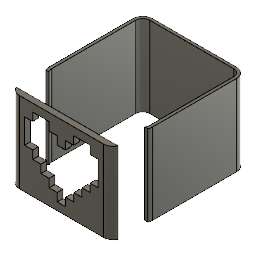
sides (Autodesk Fusion 360 design; units mm, degrees)
Autodesk Fusion 360 part; units mm, degrees
note: some values were not read from the file. Chosen so that the rebuilt part matches the saved one: which bodies a step acts on.
sketch "Sketch1" plane through (0, 0, 0) normal (0, 1, 0) x (1, 0, 0)
  line L0 (35.25, -35.25) -> (-35.25, -35.25)
  line L1 (-35.25, -35.25) -> (-35.25, 35.25)
  line L2 (-35.25, 35.25) -> (35.25, 35.25)
  line L3 (35.25, 35.25) -> (35.25, -35.25)
  line L4 (35.25, -35.25) -> (-35.25, 35.25) construction
  line L5 (-35.25, -35.25) -> (35.25, 35.25) construction
  dimension "d1" = 70.5
  dimension "d2" = 70.5
  constraint perpendicular L0 L1
  constraint parallel L0 L2
  constraint parallel L1 L3
  constraint horizontal L0
  constraint coincident L4 origin
  constraint coincident L5 origin
  measures "d1" distance of L0.end L1.end
  measures "d2" distance of L1.end L2.end
extrude "Extrude1" add sketch "Sketch1" along normal blind 2 makes body 1
sketch "Sketch2" plane through (0, 2, 0) normal (0, 1, 0) x (-1, 0, 0)
  line L0 (-35.25, -35.25) -> (35.25, -35.25)
  line L1 (35.25, -35.25) -> (35.25, 35.25)
  line L2 (35.25, 35.25) -> (-35.25, 35.25)
  line L3 (-35.25, 35.25) -> (-35.25, -35.25)
  line L4 (33.25, -33.25) -> (33.25, 33.25)
  line L5 (33.25, 33.25) -> (-33.25, 33.25)
  line L6 (-33.25, 33.25) -> (-33.25, -33.25)
  line L7 (-33.25, -33.25) -> (33.25, -33.25)
  dimension "d5" = -2
extrude "Extrude2" add sketch "Sketch2" along normal blind 55 bodies 1
fillet "Fillet1" radius 6.75 4 edges at (35.25, 28.5, 35.25) (-35.25, 28.5, 35.25) (-35.25, 28.5, -35.25) (35.25, 28.5, -35.25) on bodies 1
fillet "Fillet2" radius 4.75 4 edges at (33.25, 29.5, 33.25) (33.25, 29.5, -33.25) (-33.25, 29.5, -33.25) (-33.25, 29.5, 33.25) on bodies 1
fillet "Fillet3" radius 2 8 edges at (35.25, 0, 0) (33.273, 0, -33.273) (0, 0, -35.25) (-33.273, 0, -33.273) (-35.25, 0, 0) (-33.273, 0, 33.273) (0, 0, 35.25) (33.273, 0, 33.273) on bodies 1
sketch "Sketch3" plane through (0, 0, 0) normal (0, -1, 0) x (1, 0, 0)
  line L0 (33.25, -28.5) -> (33.25, 28.5)
  arc A0 (33.25, 28.5) -> (28.5, 33.25) centre (28.5, 28.5) ccw
  line L1 (28.5, 33.25) -> (-28.5, 33.25)
  arc A1 (-28.5, 33.25) -> (-33.25, 28.5) centre (-28.5, 28.5) ccw
  line L2 (-33.25, 28.5) -> (-33.25, -28.5)
  arc A2 (-33.25, -28.5) -> (-28.5, -33.25) centre (-28.5, -28.5) ccw
  line L3 (-28.5, -33.25) -> (28.5, -33.25)
  arc A3 (28.5, -33.25) -> (33.25, -28.5) centre (28.5, -28.5) ccw
  line L4 (-52, 44) -> (45, 44)
  line L5 (45, 44) -> (45, -37)
  line L6 (45, -37) -> (-52, -37)
  line L7 (-52, -37) -> (-52, 44)
  constraint horizontal L4
  constraint vertical L5
  constraint horizontal L6
  constraint vertical L7
extrude "Extrude3" cut sketch "Sketch3" against normal blind 2 contours L0 A0 L1 A1 L2 A2 L3 A3 | L4 L5 L6 L7 bodies 1
sketch "Sketch4" plane through (0, 0, 35.25) normal (0, 0, 1) x (1, 0, 0)
  line L0 (-28.5, 2) -> (28.5, 2)
  line L1 (28.5, 2) -> (28.5, 57)
  line L2 (28.5, 57) -> (-28.5, 57)
  line L3 (-28.5, 57) -> (-28.5, 2)
  line L4 (0, 57) -> (0, 2)
  line L5 (28.5, 29.5) -> (-28.5, 29.5)
  line L6 (0, 29.5) -> (0, 51.7)
  line L7 (0, 29.5) -> (0, 7.3)
  line L8 (0, 51.7) -> (0, 46.15)
  line L9 (0, 46.15) -> (0, 40.6)
  line L10 (0, 40.6) -> (0, 35.05)
  line L11 (0, 35.05) -> (0, 29.5)
  line L12 (0, 40.6) -> (2.775, 40.6)
  line L13 (0, 40.6) -> (-2.775, 40.6)
  line L14 (2.775, 40.6) -> (2.775, 46.15)
  line L15 (2.775, 46.15) -> (8.325, 46.15)
  line L16 (-2.775, 40.6) -> (-2.775, 46.15)
  line L17 (-2.775, 46.15) -> (-8.325, 46.15)
  line L18 (-8.325, 46.15) -> (-8.325, 51.7)
  line L19 (8.325, 46.15) -> (8.325, 51.7)
  line L20 (8.325, 51.7) -> (19.425, 51.7)
  line L21 (-8.325, 51.7) -> (-19.425, 51.7)
  line L22 (-19.425, 51.7) -> (-19.425, 46.15)
  line L23 (19.425, 51.7) -> (19.425, 46.15)
  line L24 (-19.425, 46.15) -> (-24.975, 46.15)
  line L25 (19.425, 46.15) -> (24.975, 46.15)
  line L26 (-24.975, 46.15) -> (-24.975, 29.5)
  line L27 (24.975, 46.15) -> (24.975, 29.5)
  line L28 (-24.975, 29.5) -> (-19.425, 29.5)
  line L29 (24.975, 29.5) -> (19.425, 29.5)
  line L30 (19.425, 29.5) -> (19.425, 23.95)
  line L31 (-19.425, 29.5) -> (-19.425, 23.95)
  line L32 (-19.425, 23.95) -> (-13.875, 23.95)
  line L33 (19.425, 23.95) -> (13.875, 23.95)
  line L34 (-13.875, 23.95) -> (-13.875, 18.4)
  line L35 (13.875, 23.95) -> (13.875, 18.4)
  line L36 (-13.875, 18.4) -> (-8.325, 18.4)
  line L37 (13.875, 18.4) -> (8.325, 18.4)
  line L38 (-8.325, 18.4) -> (-8.325, 12.85)
  line L39 (8.325, 18.4) -> (8.325, 12.85)
  line L40 (8.325, 12.85) -> (2.775, 12.85)
  line L41 (-8.325, 12.85) -> (-2.775, 12.85)
  line L42 (-2.775, 12.85) -> (-2.775, 7.3)
  line L43 (-2.775, 7.3) -> (2.775, 7.3)
  line L44 (2.775, 7.3) -> (2.775, 12.85)
  dimension "d13" = 22.2
  dimension "d14" = 22.2
  dimension "d17" = 5.55
  dimension "d18" = 5.55
  dimension "d19" = 2.775
  dimension "d20" = 2.775
  dimension "d21" = 5.55
  dimension "d22" = 5.55
  dimension "d23" = 5.55
  dimension "d24" = 5.55
  dimension "d25" = 11.1
  dimension "d26" = 11.1
  dimension "d27" = 5.55
  dimension "d28" = 5.55
  dimension "d29" = 5.55
  dimension "d30" = 5.55
  dimension "d31" = 16.65
  dimension "d32" = 16.65
  dimension "d33" = 5.55
  dimension "d34" = 5.55
  dimension "d35" = 5.55
  dimension "d36" = 5.55
  dimension "d37" = 5.55
  dimension "d38" = 5.55
  dimension "d39" = 5.55
  dimension "d40" = 5.55
  dimension "d41" = 5.55
  dimension "d42" = 5.55
  dimension "d43" = 5.55
  dimension "d44" = 5.55
  dimension "d45" = 5.55
  dimension "d46" = 5.55
  dimension "d47" = 5.55
  dimension "d48" = 5.55
  constraint midpoint L2 L4.start
  constraint midpoint L0 L4.end
  constraint midpoint L1 L5.start
  constraint midpoint L3 L5.end
  constraint midpoint L4 L6.start
  constraint perpendicular L5 L6
  constraint parallel L4 L7
  constraint parallel L4 L8
  constraint parallel L4 L9
  constraint parallel L6 L10
  constraint parallel L6 L11
  constraint perpendicular L9 L12
  constraint perpendicular L10 L13
  constraint perpendicular L12 L14
  constraint perpendicular L14 L15
  constraint perpendicular L13 L16
  constraint perpendicular L16 L17
  constraint perpendicular L17 L18
  constraint perpendicular L15 L19
  constraint perpendicular L19 L20
  constraint perpendicular L18 L21
  constraint perpendicular L21 L22
  constraint perpendicular L20 L23
  constraint perpendicular L22 L24
  constraint perpendicular L23 L25
  constraint perpendicular L24 L26
  constraint perpendicular L25 L27
  constraint perpendicular L26 L28
  constraint perpendicular L27 L29
  constraint perpendicular L5 L30
  constraint perpendicular L28 L31
  constraint perpendicular L31 L32
  constraint perpendicular L30 L33
  constraint perpendicular L32 L34
  constraint perpendicular L33 L35
  constraint perpendicular L34 L36
  constraint perpendicular L35 L37
  constraint perpendicular L36 L38
  constraint perpendicular L37 L39
  constraint perpendicular L39 L40
  constraint perpendicular L38 L41
  constraint perpendicular L41 L42
  constraint perpendicular L7 L43
  measures "d13" distance of L6.start L6.end
  measures "d14" distance of L6.start L7.end
  measures "d17" distance of L9.end L10.end
  measures "d18" distance of L10.end L6.start
  measures "d19" distance of L9.end L12.end
  measures "d20" distance of L9.end L13.end
  measures "d21" distance of L12.end L14.end
  measures "d22" distance of L14.end L15.end
  measures "d23" distance of L13.end L16.end
  measures "d24" distance of L16.end L17.end
  measures "d25" distance of L19.end L20.end
  measures "d26" distance of L18.end L21.end
  measures "d27" distance of L21.end L22.end
  measures "d28" distance of L20.end L23.end
  measures "d29" distance of L22.end L24.end
  measures "d30" distance of L23.end L25.end
  measures "d31" distance of L24.end L26.end
  measures "d32" distance of L25.end L27.end
  measures "d33" distance of L26.end L28.end
  measures "d34" distance of L27.end L29.end
  measures "d35" distance of L29.end L30.end
  measures "d36" distance of L28.end L31.end
  measures "d37" distance of L31.end L32.end
  measures "d38" distance of L30.end L33.end
  measures "d39" distance of L32.end L34.end
  measures "d40" distance of L33.end L35.end
  measures "d41" distance of L34.end L36.end
  measures "d42" distance of L35.end L37.end
  measures "d43" distance of L36.end L38.end
  measures "d44" distance of L37.end L39.end
  measures "d45" distance of L39.end L40.end
  measures "d46" distance of L38.end L41.end
  measures "d47" distance of L41.end L42.end
  measures "d48" distance of L42.end L43.end
extrude "Extrude5" cut sketch "Sketch4" against normal blind 0.5 from surface at -1.5 contours L4 L5 L7 L31 L32 L34 L36 L38 L41 L42 L43 | L4 L5 L7 L30 L33 L35 L37 L39 L40 L43 L44 | L4 L5 L6 L10 L11 L13 L16 L17 L18 L21 L22 L24 L26 L28 | L4 L5 L6 L10 L11 L12 L14 L15 L19 L20 L23 L25 L27 L29 bodies 1
extrude "Extrude4" cut sketch "Sketch4" against normal blind 0.5 contours L4 L5 L7 L31 L32 L34 L36 L38 L41 L42 L43 | L4 L5 L7 L30 L33 L35 L37 L39 L40 L43 L44 | L4 L5 L6 L10 L11 L13 L16 L17 L18 L21 L22 L24 L26 L28 | L4 L5 L6 L10 L11 L12 L14 L15 L19 L20 L23 L25 L27 L29 bodies 1
sketch "Sketch8" plane through (0, 0, 33.25) normal (0, 0, -1) x (-1, 0, 0)
  line L0 (2.775, 40.6) -> (2.775, 46.15)
  line L1 (2.775, 46.15) -> (8.325, 46.15)
  line L2 (8.325, 46.15) -> (8.325, 51.7)
  line L3 (8.325, 51.7) -> (19.425, 51.7)
  line L4 (19.425, 51.7) -> (19.425, 46.15)
  line L5 (19.425, 46.15) -> (24.975, 46.15)
  line L6 (24.975, 46.15) -> (24.975, 29.5)
  line L7 (24.975, 29.5) -> (19.425, 29.5)
  line L8 (19.425, 29.5) -> (19.425, 23.95)
  line L9 (19.425, 23.95) -> (13.875, 23.95)
  line L10 (13.875, 23.95) -> (13.875, 18.4)
  line L11 (13.875, 18.4) -> (8.325, 18.4)
  line L12 (8.325, 18.4) -> (8.325, 12.85)
  line L13 (8.325, 12.85) -> (2.775, 12.85)
  line L14 (2.775, 12.85) -> (2.775, 7.3)
  line L15 (2.775, 7.3) -> (-2.775, 7.3)
  line L16 (-2.775, 7.3) -> (-2.775, 12.85)
  line L17 (-2.775, 12.85) -> (-8.325, 12.85)
  line L18 (-8.325, 12.85) -> (-8.325, 18.4)
  line L19 (-8.325, 18.4) -> (-13.875, 18.4)
  line L20 (-13.875, 18.4) -> (-13.875, 23.95)
  line L21 (-13.875, 23.95) -> (-19.425, 23.95)
  line L22 (-19.425, 23.95) -> (-19.425, 29.5)
  line L23 (-19.425, 29.5) -> (-24.975, 29.5)
  line L24 (-24.975, 29.5) -> (-24.975, 46.15)
  line L25 (-24.975, 46.15) -> (-19.425, 46.15)
  line L26 (-19.425, 46.15) -> (-19.425, 51.7)
  line L27 (-19.425, 51.7) -> (-8.325, 51.7)
  line L28 (-8.325, 51.7) -> (-8.325, 46.15)
  line L29 (-8.325, 46.15) -> (-2.775, 46.15)
  line L30 (-2.775, 46.15) -> (-2.775, 40.6)
  line L31 (-2.775, 40.6) -> (2.775, 40.6)
  line L32 (28.5, 2) -> (28.5, 57)
  line L33 (28.5, 57) -> (-28.5, 57)
  line L34 (-28.5, 57) -> (-28.5, 2)
  line L35 (-28.5, 2) -> (28.5, 2)
  line L36 (28.5, 57) -> (33, 57)
  line L37 (-28.5, 57) -> (-33, 57)
  line L38 (-33, 57) -> (33, 57)
  line L39 (33, 57) -> (33, 2)
  line L40 (33, 2) -> (-33, 2)
  line L41 (-33, 2) -> (-33, 57)
  constraint coincident L32.end L33.start
  constraint perpendicular L32 L36
  constraint coincident L33.end L34.start
  constraint perpendicular L34 L37
  constraint horizontal L38
  constraint vertical L39
  constraint horizontal L40
  constraint vertical L41
extrude "Extrude12" add sketch "Sketch8" along normal blind 2 bodies 1
extrude "Extrude13" cut 1 faces at (-0.925, 25.8, 33.75) along direction (0, 0, 1) blind 41 on bodies 1 bodies 1
sketch "Sketch9" plane through (0, 0, -35.25) normal (0, 0, -1) x (-1, 0, 0)
  line L0 (-28.5, 2) -> (28.5, 2)
  line L1 (28.5, 2) -> (28.5, 57)
  line L2 (28.5, 57) -> (-28.5, 57)
  line L3 (-28.5, 57) -> (-28.5, 2)
  line L4 (0, 2) -> (0, 10)
  line L5 (6, 10) -> (-6, 10)
  line L6 (-6, 10) -> (-6, 2)
  line L7 (-6, 2) -> (6, 2)
  line L8 (6, 2) -> (6, 10)
  line L9 (6, 10) -> (-6, 2) construction
  line L10 (-6, 10) -> (6, 2) construction
  point P0 (0, 6)
  dimension "d175" = 12
  dimension "d180" = 8
  constraint midpoint L0 L4.start
  constraint perpendicular L0 L4
  constraint perpendicular L5 L6
  constraint parallel L5 L7
  constraint parallel L6 L8
  constraint horizontal L5
  constraint coincident L9 P0
  constraint coincident L10 P0
  constraint midpoint L4 P0
  measures "d175" distance of L6.end L7.end
  measures "d180" distance of L5.start L7.end
extrude "Extrude14" cut sketch "Sketch9" against normal blind 15 contours L0 L4 L5 L6 L7 | L0 L4 L5 L7 L8 bodies 1
sketch "Sketch10" plane through (0, 0, 31.25) normal (0, 0, -1) x (-1, 0, 0)
  line L0 (-2.775, 46.15) -> (-2.775, 40.6)
  line L1 (-2.775, 40.6) -> (2.775, 40.6)
  line L2 (2.775, 40.6) -> (2.775, 46.15)
  line L3 (2.775, 46.15) -> (8.325, 46.15)
  line L4 (8.325, 46.15) -> (8.325, 51.7)
  line L5 (8.325, 51.7) -> (19.425, 51.7)
  line L6 (19.425, 51.7) -> (19.425, 46.15)
  line L7 (19.425, 46.15) -> (24.975, 46.15)
  line L8 (24.975, 46.15) -> (24.975, 29.5)
  line L9 (24.975, 29.5) -> (19.425, 29.5)
  line L10 (19.425, 29.5) -> (19.425, 23.95)
  line L11 (19.425, 23.95) -> (13.875, 23.95)
  line L12 (13.875, 23.95) -> (13.875, 18.4)
  line L13 (13.875, 18.4) -> (8.325, 18.4)
  line L14 (8.325, 18.4) -> (8.325, 12.85)
  line L15 (8.325, 12.85) -> (2.775, 12.85)
  line L16 (2.775, 12.85) -> (2.775, 7.3)
  line L17 (2.775, 7.3) -> (-2.775, 7.3)
  line L18 (-2.775, 7.3) -> (-2.775, 12.85)
  line L19 (-2.775, 12.85) -> (-8.325, 12.85)
  line L20 (-8.325, 12.85) -> (-8.325, 18.4)
  line L21 (-8.325, 18.4) -> (-13.875, 18.4)
  line L22 (-13.875, 18.4) -> (-13.875, 23.95)
  line L23 (-13.875, 23.95) -> (-19.425, 23.95)
  line L24 (-19.425, 23.95) -> (-19.425, 29.5)
  line L25 (-19.425, 29.5) -> (-24.975, 29.5)
  line L26 (-24.975, 29.5) -> (-24.975, 46.15)
  line L27 (-24.975, 46.15) -> (-19.425, 46.15)
  line L28 (-19.425, 46.15) -> (-19.425, 51.7)
  line L29 (-19.425, 51.7) -> (-8.325, 51.7)
  line L30 (-8.325, 51.7) -> (-8.325, 46.15)
  line L31 (-8.325, 46.15) -> (-2.775, 46.15)
  line L32 (-32.373, 57) -> (-32.373, 2)
  line L33 (-32.373, 2) -> (32.373, 2)
  line L34 (32.373, 2) -> (32.373, 57)
  line L35 (32.373, 57) -> (-32.373, 57)
  line L36 (-46.9699, 79.9985) -> (58.499, 79.9985)
  line L37 (58.499, 79.9985) -> (58.499, -18.9089)
  line L38 (58.499, -18.9089) -> (-46.9699, -18.9089)
  line L39 (-46.9699, -18.9089) -> (-46.9699, 79.9985)
  constraint horizontal L36
  constraint vertical L37
  constraint horizontal L38
  constraint vertical L39
extrude "Extrude15" cut sketch "Sketch10" along normal blind 0.0001 contours L32 L33 L34 L35 | L36 L37 L38 L39 bodies 1 makes body 2 at (31.4346, 29.5, 31.25)
move_body "Move1" bodies 2 to x (1, 0, 0) y (0, 1, 0) z (0, 0, 1) at (0, 0, 20)
equation "d13 = ( 44.4 / 2 ) * 1 mm"
equation "d14 = ( 44.4 / 2 ) * 1 mm"
equation "d19 = ( 5.55 / 2 ) * 1 mm"
equation "d20 = ( 5.55 / 2 ) * 1 mm"
equation "d25 = ( 5.55 * 2 ) * 1 mm"
equation "d26 = ( 5.55 * 2 ) * 1 mm"
equation "d31 = ( 5.55 * 3 ) * 1 mm"
equation "d32 = ( 5.55 * 3 ) * 1 mm"
